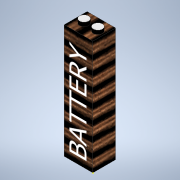
# Autodesk Inventor part: battery
Saved by Autodesk Inventor 2021 (Build 250183000, 183)
## iProperties
Created: 2021-08-02
Part Number: battery
Material: Generic
Document SubType Name: Modeling
Designer: Dell
Density: 1 g/cm^3
Appearance: Default
Author: Dell
Autodesk Inventor part; units mm, degrees
ref_plane "YZ Plane" through (0, 0, 0) normal (1, 0, 0) x (0, 1, 0)
ref_plane "XZ Plane" through (0, 0, 0) normal (0, 1, 0) x (-1, 0, 0)
ref_plane "XY Plane" through (0, 0, 0) normal (0, 0, 1) x (1, 0, 0)
sketch "Sketch1" plane through (0, 0, 0) normal (0, 1, 0) x (-1, 0, 0)
  line L0 (0.035, -1.4579) -> (15.035, -1.4579)
  line L1 (15.035, -1.4579) -> (15.035, -13.4579)
  line L2 (15.035, -13.4579) -> (0.035, -13.4579)
  line L3 (0.035, -13.4579) -> (0.035, -1.4579)
  point P0 (0, 0)
  dimension "d0" = 12
  dimension "d1" = 15
  constraints: 8 end point, 2 parallel, 1 horizontal, 1 perpendicular
  measures "d0" distance of L0.end L1.end
  measures "d1" distance of L1.end L2.end
extrude "Extrusion1" add sketch "Sketch1" along normal blind 60
sketch "Sketch2" plane through (0, 60, 0) normal (0, 1, 0) x (1, 0, 0)
  circle A0 centre (-10.626, 7.4579) radius 2.3855
  circle A1 centre (-3.3773, 7.4579) radius 2.3855
  point P0 (0, 0)
  constraints: 2 centre point
extrude "Extrusion2" add sketch "Sketch2" along normal blind 2
sketch "Sketch3" plane through (-15.035, 0, -1.4579) normal (0, 0, 1) x (1, 0, 0)
  line L0 (2.6785, 2.7506) -> (2.6785, 53.826) construction
  line L1 (2.6785, 53.826) -> (11.6785, 53.826) construction
  line L2 (11.6785, 53.826) -> (11.6785, 2.7506) construction
  line L3 (11.6785, 2.7506) -> (2.6785, 2.7506) construction
  point P0 (15.035, 0)
  dimension "d2" = 60
  dimension "d3" = 0
  constraints: 2 other
body "Solid1"
